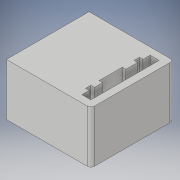
# Autodesk Inventor part: rear_light_mount
Saved by Autodesk Inventor 2019 (Build 230136000, 136)
## iProperties
Created: 2019-09-25
Part Number: rear_light_mount
Material: Generic
Document SubType Name: Modeling
Designer: Alex
Density: 1 g/cm^3
Appearance: Default
Author: Alex
Autodesk Inventor part; units mm, degrees
ref_plane "YZ Plane" through (0, 0, 0) normal (1, 0, 0) x (0, 1, 0)
ref_plane "XZ Plane" through (0, 0, 0) normal (0, 1, 0) x (-1, 0, 0)
ref_plane "XY Plane" through (0, 0, 0) normal (0, 0, 1) x (1, 0, 0)
sketch "Sketch1" plane through (0, 0, 0) normal (0, 1, 0) x (-1, 0, 0)
  line L0 (0, 0) -> (2.5, 0)
  line L1 (2.5, -19) -> (0, -19)
  line L2 (0, -19) -> (0, 0)
  line L3 (11.5, 2) -> (-1, 2)
  line L4 (-2, 1) -> (-2, -20)
  line L5 (-1, -21) -> (11.5, -21)
  line L6 (2.5, -2) -> (3.5, -2)
  line L7 (2.5, -17) -> (3.5, -17)
  line L8 (3.5, -2) -> (3.5, -3.5)
  line L9 (3.5, -3.5) -> (2.5, -3.5)
  line L10 (3.5, -17) -> (3.5, -15.5)
  line L11 (3.5, -15.5) -> (2.5, -15.5)
  line L12 (2.5, -2) -> (2.5, 0)
  line L13 (2.5, -3.5) -> (2.5, -15.5)
  line L14 (2.5, -17) -> (2.5, -19)
  arc A0 (-1, 2) -> (-2, 1) centre (-1, 1) ccw
  arc A1 (-2, -20) -> (-1, -21) centre (-1, -20) ccw
  line L15 (11.5, 2) -> (21.5, 2)
  line L16 (11.5, -21) -> (21.5, -21)
  line L17 (21.5, -21) -> (21.5, 2)
  dimension "d0" = 19
  dimension "d1" = 2.5
  dimension "d3" = 2
  dimension "d4" = 2
  dimension "d5" = 2
  dimension "d7" = 1
  dimension "d8" = 15
  dimension "d10" = 1.5
  dimension "d11" = 1.5
  dimension "d12" = 1
  dimension "d21" = 10
  dimension "d22" = 4
  constraints: 36 end point, 5 horizontal, 4 point on circle, 4 tangent, 2 centre point, 2 collinear, 2 parallel, 2 perpendicular, 2 vertical, 1 equal radius, 1 point on line
  measures "d0" distance of L0.end L1.start
  measures "d1" distance of L1.start L1.end
  measures "d3" distance between parallel lines of L4 L2
  measures "d4" distance between parallel lines of L3 L0
  measures "d5" distance between parallel lines of L5 L1
  measures "d7" distance of L6.start L6.end
  measures "d8" distance between parallel lines of L7 L6
  measures "d10" distance of L6.end L8.end
  measures "d11" distance of L7.end L10.end
  measures "d12" radius of A0
  measures "d21" distance of L3.start L15.end
  measures "d22" distance between parallel lines of L5 L7
extrude "Extrusion1" add sketch "Sketch1" along normal blind 14.5
sketch "Sketch5" plane through (0, 14.5, 0) normal (0, 1, 0) x (1, 0, 0)
  line L0 (-2.5, 5.75) -> (-3.5, 5.75)
  line L1 (-3.5, 5.75) -> (-3.5, 12.25)
  line L2 (-3.5, 12.25) -> (-2.5, 12.25)
  line L3 (-2.5, 12.25) -> (-2.5, 5.75)
  line L4 (-2.5, 3.5) -> (-2.5, 15.5) projected
  line L5 (-21.5, -2) -> (1, -2) projected
  point P0 (0, 0)
  point P1 (-11.5, -2)
  dimension "d15" = 1
  dimension "d16" = 6.5
  dimension "d17" = 0
  dimension "d18" = 7.75
  constraints: 8 end point, 2 parallel, 1 horizontal, 1 perpendicular
  measures "d15" distance between parallel lines of L1 L3
  measures "d16" distance between parallel lines of L2 L0
  measures "d17" distance between parallel lines of L4 L3
  measures "d18" distance between parallel lines of L5 L0
extrude "Extrusion2" cut sketch "Sketch5" against normal blind 13
body "Solid1"
